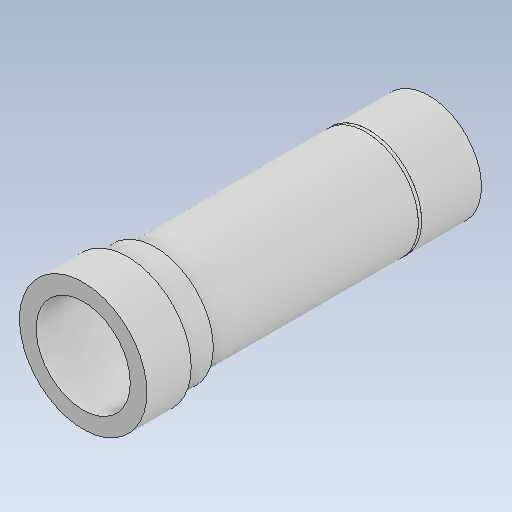
# Autodesk Inventor part: atraktos_eisodou
Saved by Autodesk Inventor 2021 (Build 250183000, 183)
## iProperties
Created: 2020-12-26
Part Number: atraktos_eisodou
Material: Generic
Document SubType Name: Modeling
Designer: Angelos
Density: 1 g/cm^3
Appearance: Default
Author: Angelos
Autodesk Inventor part; units mm, degrees
ref_plane "YZ Plane" through (0, 0, 0) normal (1, 0, 0) x (0, 1, 0)
sketch "Sketch1" plane through (0, 0, 0) normal (0, 0, 1) x (1, 0, 0)
  circle A0 centre (0, 0) radius 45
  line L0 (-2.0617, 37.7437) -> (1.1161, 37.7437) construction
  line L1 (-2.0617, 37.7437) -> (1.8744, 37.7437) construction
  line L2 (-2.0617, 37.7437) -> (-2.1753, 36.936)
  line L3 (2.0617, 37.7437) -> (2.1753, 36.936)
  line L4 (-2.0617, 37.7437) -> (-1.75, 39.9617)
  line L5 (2.0617, 37.7437) -> (1.75, 39.9617)
  line L6 (0, 0) -> (0, 11.2852)
  circle A1 centre (0, 0) radius 37
  circle A2 centre (0, 0) radius 40
  dimension "d1" = 80
  dimension "d6" = 74
  dimension "d0" = 90
  dimension "d2" = 0
  dimension "d3" = 0
  dimension "d4" = 0
  dimension "d5" = 0
  dimension "d7" = 82
  dimension "d8" = 36.936
  dimension "d9" = 2.1753
  dimension "d10" = 2.0617
  dimension "d11" = 11.2852
  constraints: 14 end point, 3 symmetric about line, 2 coincident, 2 horizontal, 1 centre point, 1 vertical, 6 other
  measures "d0" diameter of A0
  measures "d2" distance of point (0, 0) point (0, 0)
  measures "d3" distance of point (0, 0) point (0, 0)
  measures "d4" distance of point (0, 0) point (0, 0)
  measures "d5" distance of point (0, 0) point (0, 0)
  measures "d7" angle of L0 L4
  measures "d8" vertical distance of point (0, 0) L2.end
  measures "d9" horizontal distance of point (0, 0) L2.end
  measures "d10" horizontal distance of point (0, 0) L2.start
  measures "d11" distance of L6.start L6.end
extrude "Extrusion2" add sketch "Sketch1" along normal blind 10 contours L4 A2 L5 L3 A1 L2 | L2 A1 L3 L5 A2 L4
fillet "Fillet1" radius 3 2 edges at (2.1753, -36.936, 0) (2.1753, -36.936, 10)
extrude "Extrusion3" cut sketch "Sketch1" along normal through all contours L4 A2 L5 L3 A1 L2 picked at (-0.1945, 37.9938)
pattern_circular "Circular Pattern1" count 36 over 360 about axis through (0, 0, -10) along (0, 0, 1) of "Extrusion3"
extrude "Extrusion9" add sketch "Sketch1" along normal blind 10
sketch "Sketch7" plane through (0, 0, 10) normal (0, 0, 1) x (1, 0, 0)
  circle A0 centre (0, 0) radius 45
  circle A1 centre (0, 0) radius 42.5
  dimension "d51" = 90
  dimension "d52" = 85
  constraints: 2 centre point, 2 coincident
  measures "d51" diameter of A0
  measures "d52" diameter of A1
extrude "Extrusion10" add sketch "Sketch7" along normal blind 29.94
ref_plane "Work Plane5" through (0, 0, 42.94) normal (0, 0, 1) x (1, 0, 0)
ref_plane "Work Plane6" through (0, 0, 42.94) normal (0, 0, 1) x (1, 0, 0)
sketch "Sketch11" plane through (0, 0, 42.94) normal (0, 0, 1) x (1, 0, 0)
  circle A0 centre (0, 0) radius 47.5
  circle A1 centre (0, 0) radius 42.5
  dimension "d68" = 95
  dimension "d69" = 85
  constraints: 2 centre point, 2 coincident
  measures "d68" diameter of A0
  measures "d69" diameter of A1
extrude "Extrusion14" add sketch "Sketch11" along normal blind 190
sketch "Sketch15" plane through (0, 0, 232.94) normal (0, 0, 1) x (1, 0, 0)
  circle A0 centre (0, 0) radius 42.5
  circle A1 centre (0, 0) radius 52.5
  dimension "d78" = 85
  dimension "d79" = 105
  constraints: 2 centre point, 2 coincident
  measures "d78" diameter of A0
  measures "d79" diameter of A1
extrude "Extrusion16" add sketch "Sketch15" along normal blind 25
sketch "Sketch16" plane through (0, 0, 257.94) normal (0, 0, 1) x (1, 0, 0)
  circle A0 centre (0, 0) radius 42.5
  circle A1 centre (0, 0) radius 57.5
  dimension "d82" = 85
  dimension "d83" = 115
  constraints: 2 centre point, 2 coincident
  measures "d82" diameter of A0
  measures "d83" diameter of A1
extrude "Extrusion17" add sketch "Sketch16" along normal blind 40
sketch "Sketch18" plane through (0, 0, 42.94) normal (0, 0, -1) x (-1, 0, 0)
  circle A0 centre (0, 0) radius 45
  circle A1 centre (0, 0) radius 47.5
  dimension "d86" = 90
  dimension "d87" = 95
  constraints: 2 centre point, 2 coincident
  measures "d86" diameter of A0
  measures "d87" diameter of A1
extrude "Extrusion19" add sketch "Sketch18" along normal blind 57.07
sketch "Sketch19" plane through (0, 0, 42.94) normal (0, 0, 1) x (1, 0, 0)
  circle A0 centre (0, 0) radius 42.5
  circle A1 centre (0, 0) radius 47.5436
  constraints: 2 centre point, 2 coincident
extrude "Extrusion20" add sketch "Sketch19" against normal blind 3
body "Solid1"
